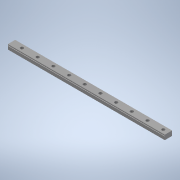
# Autodesk Inventor part: Stand
Saved by Autodesk Inventor 2021.3 (Build 253353000, 353)
## iProperties
Created: 2021-06-01
Part Number: Stand
Material: Steel, Wrought
Document SubType Name: Modeling
Designer: vivek
Density: 7.85 g/cm^3
Appearance: Steel
Author: vivek
Autodesk Inventor part; units mm, degrees
ref_plane "YZ Plane" through (0, 0, 0) normal (1, 0, 0) x (0, 1, 0)
ref_plane "XZ Plane" through (0, 0, 0) normal (0, 1, 0) x (-1, 0, 0)
ref_plane "XY Plane" through (0, 0, 0) normal (0, 0, 1) x (1, 0, 0)
sketch "Sketch1" plane through (0, 0, 0) normal (0, 0, 1) x (1, 0, 0)
  line L0 (150, -7) -> (-150, -7)
  line L1 (-150, -7) -> (-150, 7)
  line L2 (-150, 7) -> (150, 7)
  line L3 (150, 7) -> (150, -7)
  line L4 (0, 0) -> (0, 3.6651)
  line L5 (0, 0) -> (24.411, 0)
  point P0 (0, 7)
  point P1 (150, 0)
  dimension "d0" = 300
  dimension "d1" = 14
  constraints: 12 end point, 3 parallel, 2 midpoint, 2 perpendicular, 2 point on line, 1 horizontal
  measures "d0" distance of L1.end L2.end
  measures "d1" distance of L0.end L1.end
extrude "Extrusion1" add sketch "Sketch1" along normal blind 9
sketch "Sketch2" plane through (-150, -7, 0) normal (-1, 0, 0) x (0, 0, 1)
  line L0 (0, 14) -> (9, 14) projected
  line L1 (6.5, 13.134) -> (6, 14)
  line L2 (6, 14) -> (7, 14)
  line L3 (7, 14) -> (6.5, 13.134)
  point P0 (0, 7)
  point P1 (6.5, 13.7113)
  dimension "d4" = 1
  dimension "d5" = 2
  constraints: 6 end point, 1 collinear, 7 other
  measures "d4" distance of L2.end L1.start
  measures "d5" distance of L0.end L2.end
extrude "Extrusion2" cut sketch "Sketch2" against normal through all
mirror "Mirror1" about plane through (0, 0, 0) normal (0, 1, 0) of "Extrusion2"
sketch "Sketch3" plane through (0, 0, 9) normal (0, 0, 1) x (1, 0, 0)
  line L0 (-150, 7) -> (-150, -7) projected
  circle A0 centre (-130, 0) radius 3
  point P0 (0, 0)
  dimension "d9" = 6
  dimension "d10" = 20
  constraints: 1 centre point
  measures "d9" diameter of A0
  measures "d10" distance from line of L0 A0.centre
extrude "Extrusion3" cut sketch "Sketch3" against normal through all
pattern_linear "Rectangular Pattern1" count 10 spacing 30 along (1, 0, 0) of "Extrusion3"
ref_plane "Work Plane1" through (0, 0, 0) normal (0, 1, 0) x (-1, 0, 0)
body "Solid1"
